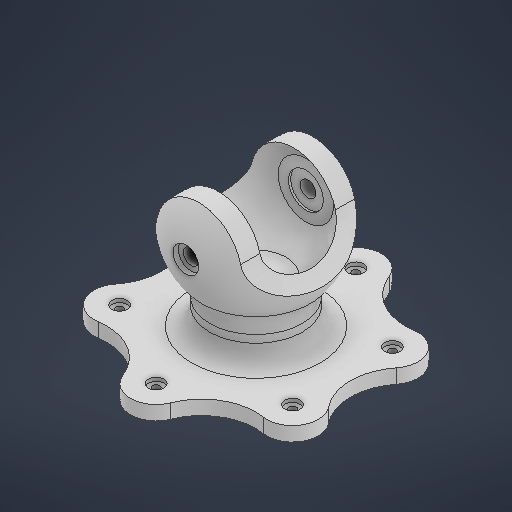
# Autodesk Inventor part: b5
Saved by Autodesk Inventor 2025.4 (Build 294407000, 407)
## iProperties
Created: 2026-05-19
Part Number: b5
Material: Generic
Document SubType Name: Modeling
Designer: VuQuan
Density: 1 g/cm^3
Appearance: Default
Author: VuQuan
Autodesk Inventor part; units mm, degrees
note: some values were not read from the file. Chosen so that the rebuilt part matches the saved one: copy form of "Mirror2".
ref_plane "YZ Plane" through (0, 0, 0) normal (1, 0, 0) x (0, 1, 0)
sketch "Sketch1" plane through (0, 0, 0) normal (0, 1, 0) x (-1, 0, 0)
  line L0 (0, 140) -> (0, -140) construction
  line L1 (140, 0) -> (-140, 0) construction
  arc A0 (0, -140) -> (0, 140) centre (0, 0) ccw construction
  arc A1 (149.3461, 47.5) -> (149.346, -47.5) centre (208.6735, 0) ccw
  circle A2 centre (121.2436, -70) radius 5
  circle A3 centre (121.2436, -70) radius 11
  circle A4 centre (121.2436, -70) radius 17.5
  line L2 (121.2436, -70) -> (0, 0) construction
  arc A5 (115.8092, -105.5875) -> (149.346, -47.5) centre (121.2436, -70) ccw
  circle A6 centre (0, 0) radius 32
  circle A7 centre (0, 0) radius 60
  circle A8 centre (0, 0) radius 76
  arc A9 (149.3461, 47.5) -> (115.8092, 105.5875) centre (121.2436, 70) ccw
  arc A10 (33.5368, 153.0875) -> (115.8092, 105.5875) centre (104.3368, 180.7166) ccw
  arc A11 (33.5368, 153.0875) -> (-33.5368, 153.0875) centre (0, 140) ccw
  arc A12 (-115.8092, 105.5875) -> (-33.5368, 153.0875) centre (-104.3368, 180.7166) ccw
  arc A13 (-115.8092, 105.5875) -> (-149.346, 47.5) centre (-121.2436, 70) ccw
  arc A14 (-149.3461, -47.5) -> (-149.346, 47.5) centre (-208.6735, 0) ccw
  arc A15 (-149.3461, -47.5) -> (-115.8092, -105.5875) centre (-121.2436, -70) ccw
  arc A16 (-33.5368, -153.0875) -> (-115.8092, -105.5875) centre (-104.3368, -180.7166) ccw
  arc A17 (-33.5368, -153.0875) -> (33.5368, -153.0875) centre (0, -140) ccw
  arc A18 (115.8092, -105.5875) -> (33.5368, -153.0875) centre (104.3368, -180.7166) ccw
  point P0 (33.5368, 153.0875)
  point P1 (-115.8092, 105.5875)
  point P2 (-149.3461, -47.5)
  point P3 (-33.5368, -153.0875)
  point P4 (115.8092, -105.5875)
  point P5 (149.3461, 47.5)
  dimension "d0" = 140
  dimension "d1" = 10
  dimension "d2" = 22
  dimension "d3" = 35
  dimension "d4" = 60
  dimension "d5" = 36
  dimension "d6" = 76
  dimension "d11" = 64
  dimension "d12" = 120
  dimension "d13" = 152
  dimension "d18" = 360
  constraints: 28 point on circle, 19 centre point, 8 coincident, 6 end point, 3 point on line, 2 midpoint, 1 horizontal, 1 perpendicular, 1 tangent, 1 vertical, 43 other
  measures "d0" radius of A0
  measures "d1" diameter of A2
  measures "d2" diameter of A3
  measures "d3" diameter of A4
  measures "d4" angle of L0 L2
  measures "d5" radius of A5
  measures "d6" radius of A1
  measures "d11" diameter of A6
  measures "d12" diameter of A7
  measures "d13" diameter of A8
extrude "Extrusion1" add sketch "Sketch1" along normal blind 20 contours A1 A5 A18 A17 A16 A15 A14 A13 A12 A11 A10 A9 | A2 | A3 | A4 | A6 | A7 | A8
extrude "Extrusion2" cut sketch "Sketch1" along normal blind 2 contours A2 | A3 | A4
extrude "Extrusion3" cut sketch "Sketch1" against normal blind 5 from surface at 20 contours A3
extrude "Extrusion5" cut sketch "Sketch1" along normal up to surface (20 mm away) contours A2
pattern_circular "Circular Pattern2" count 6 over 360 about axis through (0, -10, 0) along (0, 1, 0) of "Extrusion5", "Extrusion3", "Extrusion2"
sketch "Sketch2" plane through (0, 0, 0) normal (0, 0, 1) x (1, 0, 0)
  line L0 (0, 0) -> (0, 256)
  arc A0 (-80, 210) -> (-65, 74.0066) centre (0, 150) ccw
  line L1 (-65, 0) -> (-65, 74.0066)
  line L2 (0, 82.2228) -> (-42.5, 82.2228)
  arc A1 (-52.915, 210) -> (-42.5, 82.2228) centre (0, 150) ccw
  line L3 (-52.915, 210) -> (-80, 210)
  line L4 (-65, 0) -> (0, 0)
  dimension "d38" = 100
  dimension "d39" = 150
  dimension "d40" = 80
  dimension "d41" = 85
  dimension "d63" = 130
  dimension "d64" = 60
  constraints: 10 end point, 4 point on circle, 3 horizontal, 2 centre point, 2 coincident, 2 horizontal alignment, 2 point on line, 2 vertical
  measures "d38" radius of A0
  measures "d39" distance of point (0, 0) A0.centre
  measures "d40" radius of A1
  measures "d41" diameter of L2.end L0
  measures "d63" diameter of L1 L0
  measures "d64" distance from line of A0.centre L3
revolve "Revolution1" add sketch "Sketch2" angle 360 about axis through (0, 0, 0) along (0, 1, 0)
sketch "Sketch3" plane through (0, 0, 0) normal (0, 0, 1) x (1, 0, 0)
  line L0 (80, 210) -> (-80, 210) projected
  arc A0 (-80, 210) -> (80, 210) centre (0, 150) ccw projected
  arc A1 (45.8258, 188.7298) -> (-58.4116, 163.7143) centre (0, 150) ccw
  arc A2 (-93.461, 114.4326) -> (-58.4116, 163.7143) centre (-136.2938, 182) ccw
  line L1 (0, 0) -> (0, 210) construction
  arc A3 (58.4116, 163.7143) -> (45.8258, 188.7298) centre (0, 150) ccw
  arc A4 (58.4116, 163.7143) -> (93.461, 114.4326) centre (136.2938, 182) ccw
  line L2 (93.461, 114.4326) -> (136.2938, 114.4326)
  line L3 (136.2938, 114.4326) -> (136.2938, 250)
  line L4 (136.2938, 250) -> (-136.2938, 250)
  line L5 (-136.2938, 250) -> (-136.2938, 114.4326)
  line L6 (-136.2938, 114.4326) -> (-93.461, 114.4326)
  dimension "d44" = 60
  dimension "d45" = 80
  dimension "d46" = 182
  constraints: 12 end point, 10 point on circle, 4 centre point, 4 symmetric about line, 3 perpendicular, 3 point on line, 2 tangent, 1 coincident, 1 horizontal, 1 vertical, 2 other
  measures "d44" radius of A1
  measures "d45" radius of A2
  measures "d46" vertical distance of A2.centre L1.start
extrude "Extrusion6" cut sketch "Sketch3" along normal through all both and the other way through all contours A0 A4 A3 A1 L0 | L0 A0 L6 L5 L4 L3 L2 | A1 A2 A0 L0
ref_plane "Work Plane1" through (0, 0, -70) normal (0, 0, 1) x (1, 0, 0)
sketch "Sketch5" plane through (0, 0, -70) normal (0, 0, 1) x (1, 0, 0)
  circle A0 centre (0, 150) radius 38.7298
  point P0 (0, 0)
  constraints: 1 centre point, 1 coincident
extrude "Extrusion7" add sketch "Sketch5" against normal blind 10
mirror "Mirror1" about plane through (0, 0, 0) normal (0, 0, 1) of "Extrusion7"
ref_plane "Work Plane2" through (0, 0, -91) normal (0, 0, 1) x (1, 0, 0)
sketch "Sketch4" plane through (0, 0, 0) normal (0, 0, 1) x (1, 0, 0)
  arc A0 (58.4116, 163.7143) -> (-58.4116, 163.7143) centre (0, 150) ccw projected
  circle A1 centre (0, 150) radius 18
  circle A2 centre (0, 150) radius 24.5
  circle A3 centre (0, 150) radius 11
  point P0 (0, 0)
  point P1 (-45.8258, 188.7298)
  dimension "d49" = 36
  dimension "d50" = 49
  dimension "d51" = 22
  constraints: 3 centre point, 3 coincident
  measures "d49" diameter of A1
  measures "d50" diameter of A2
  measures "d51" diameter of A3
extrude "Extrusion8" cut sketch "Sketch4" against normal blind 73 contours A1 | A2 | A3
extrude "Extrusion9" cut sketch "Sketch4" against normal up to next from surface at -91 contours A1 | A3
extrude "Extrusion10" cut sketch "Sketch4" against normal through all contours A3
mirror "Mirror2" about plane through (0, 0, 0) normal (0, 0, 1) of "Extrusion8", "Extrusion9", "Extrusion10" geometry pattern yes
fillet "Fillet1" radius 25 1 edges at (65, 20, 0)
fillet "Fillet2" radius 45 1 edges at (65, 74.0066, 0)
body "Solid1"
